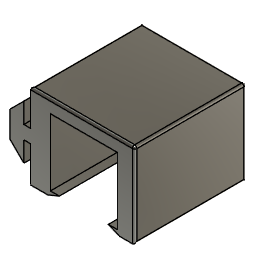
light bracket v2 (Autodesk Fusion 360 design; units mm, degrees)
Autodesk Fusion 360 part; units mm, degrees
sketch "Sketch1" plane through (0, 0, 0) normal (0, 0, 1) x (1, 0, 0) in component "Light Braccket"
  line L0 (0, 0) -> (-25, 0)
  line L1 (-25, 0) -> (-25, 25)
  line L2 (-25, 25) -> (0, 25)
  line L3 (0, 25) -> (0, 0)
  dimension "d1" = 25
  dimension "d2" = 25
  constraint horizontal L0
  constraint vertical L1
  constraint horizontal L2
  constraint vertical L3
  constraint coincident L0.start L3.end
  measures "d1" distance of L0.start L0.end
  measures "d2" distance of L0.start L2.end
extrude "Extrude1" add sketch "Sketch1" along normal blind 25 in component "Light Braccket"
sketch "Sketch2" plane through (0, 0, 0) normal (0, -1, 0) x (1, 0, 0) in component "Light Braccket"
  line L0 (-25, 0) -> (0, 0)
  line L1 (0, 0) -> (0, 25)
  line L2 (0, 25) -> (-25, 25)
  line L3 (-25, 25) -> (-25, 0)
  line L4 (-0.3536, 0) -> (-2.9142, 1.0607)
  line L5 (-0.3536, 0) -> (0.9236, 0) construction
  line L6 (-2.9142, 1.0607) -> (-0.9142, 1.0607)
  line L7 (-0.9142, 1.0607) -> (-0.9142, 16.0607)
  line L8 (-0.9142, 18.8102) -> (-15.9142, 18.8102) construction
  line L9 (-8.4142, 18.8102) -> (-8.4142, -0.114) construction
  line L10 (-16.4749, 0) -> (-13.9142, 1.0607)
  line L11 (-13.9142, 1.0607) -> (-15.9142, 1.0607)
  line L12 (-15.9142, 1.0607) -> (-15.9142, 16.0607)
  line L13 (-0.9142, 16.0607) -> (-15.9142, 16.0607)
  dimension "d14" = 15
  constraint horizontal L5
  constraint horizontal L6
  constraint perpendicular L6 L7
  constraint coincident L7 L8.start
  constraint perpendicular L7 L8
  constraint midpoint L8 L9.start
  constraint perpendicular L0 L9
  constraint symmetric L4.start L9 L10.start
  constraint symmetric L4.end L9 L10.end
  constraint symmetric L6.end L9 L11.end
  constraint symmetric L7.end L9 L12.end
  constraint perpendicular L12 L13
  measures "d14" distance of L8.start L8.end
extrude "Extrude2" cut sketch "Sketch2" against normal blind 40 contours L0 L4 L6 L7 L10 L11 L12 L13 in component "Light Braccket"
sketch "Sketch3" plane through (0, 0, 0) normal (0, -1, 0) x (1, 0, 0) in component "Light Braccket"
  line L0 (-16.4749, 0) -> (-13.9142, 1.0607)
  line L1 (-13.9142, 1.0607) -> (-15.9142, 1.0607)
  line L2 (-15.9142, 1.0607) -> (-15.9142, 16.0607)
  line L3 (-15.9142, 16.0607) -> (-0.9142, 16.0607)
  line L4 (-0.9142, 16.0607) -> (-0.9142, 1.0607)
  line L5 (-0.9142, 1.0607) -> (-2.9142, 1.0607)
  line L6 (-2.9142, 1.0607) -> (-0.3536, 0)
  line L7 (-0.3536, 0) -> (0, 0)
  line L8 (0, 0) -> (0, 25)
  line L9 (0, 25) -> (-25, 25)
  line L10 (-25, 25) -> (-25, 0)
  line L11 (-25, 0) -> (-16.4749, 0)
  line L12 (-25, 25) -> (0, 25)
  line L13 (0, 25) -> (0, 19)
  line L14 (0, 19) -> (-25, 19)
  line L15 (-25, 19) -> (-25, 25)
  constraint horizontal L12
  constraint vertical L13
  constraint horizontal L14
  constraint vertical L15
  constraint coincident L8 L13.end
  constraint coincident L9.end L10.start
extrude "Extrude3" cut sketch "Sketch3" against normal blind 39 contours L8 L9 L10 L12 L13 L14 L15 in component "Light Braccket"
sketch "Sketch4" plane through (0, 0, 0) normal (0, -1, 0) x (1, 0, 0) in component "Light Braccket"
  line L0 (0, 19) -> (-25, 19)
  line L1 (-25, 19) -> (-25, 0)
  line L2 (-25, 0) -> (-16.4749, 0)
  line L3 (-16.4749, 0) -> (-13.9142, 1.0607)
  line L4 (-13.9142, 1.0607) -> (-15.9142, 1.0607)
  line L5 (-15.9142, 1.0607) -> (-15.9142, 16.0607)
  line L6 (-15.9142, 16.0607) -> (-0.9142, 16.0607)
  line L7 (-0.9142, 16.0607) -> (-0.9142, 1.0607)
  line L8 (-0.9142, 1.0607) -> (-2.9142, 1.0607)
  line L9 (-2.9142, 1.0607) -> (-0.3536, 0)
  line L10 (-0.3536, 0) -> (0, 0)
  line L11 (0, 0) -> (0, 19)
  line L12 (-25, 0) -> (-25, 6.6)
  line L13 (-25, 6.6) -> (-21.8712, 3.4712)
  line L14 (-25, 6.6) -> (-20.5752, 6.6) construction
  line L15 (-21.8712, 3.4712) -> (-21.8712, 8)
  line L16 (-21.8712, 8) -> (-20.3712, 8)
  line L17 (-20.3712, 8) -> (-20.3712, 0)
  line L18 (-25, 0) -> (-20.3712, 0)
  line L19 (-25, 9.5) -> (0, 9.5) construction
  line L20 (-25, 12.4) -> (-21.8712, 15.5288)
  line L21 (-21.8712, 15.5288) -> (-21.8712, 11)
  line L22 (-20.3712, 11) -> (-20.3712, 19)
  line L23 (-21.8712, 11) -> (-20.3712, 11)
  line L24 (-25, 19) -> (-20.3712, 19)
  line L25 (-25, 19) -> (-25, 12.4)
  dimension "d19" = 6.6
  dimension "d20" = 45
  dimension "d21" = 1.5
  constraint coincident L1.end L2.start
  constraint perpendicular L0 L12
  constraint horizontal L14
  constraint perpendicular L14 L15
  constraint perpendicular L15 L16
  constraint coincident L2 L17.end
  constraint perpendicular L2 L17
  constraint midpoint L1 L19.start
  constraint midpoint L11 L19.end
  constraint symmetric L1.end L19 L0.end
  constraint symmetric L12.end L19 L20.start
  constraint symmetric L13.end L19 L20.end
  constraint symmetric L15.end L19 L21.end
  constraint symmetric L16.end L19 L22.start
  constraint symmetric L17.end L19 L22.end
  measures "d19" distance of L1.end L12.end
  measures "d20" angle of L13 L14
  measures "d21" distance of L15.end L16.end
extrude "Extrude4" cut sketch "Sketch4" against normal blind 33.5 contours L0 L1 L20 L21 L22 L23 L24 L25 | L1 L2 L12 L13 L15 L16 L17 L18 in component "Light Braccket"
sketch "Sketch1 (2)" plane through (0, 0, 0) normal (1, 0, 0) x (0, 1, 0)
  line L0 (25, 19) -> (0, 19)
  line L1 (0, 19) -> (0, 0)
  line L2 (0, 0) -> (25, 0)
  line L3 (25, 0) -> (25, 19)
extrude "Extrude5" add sketch "Sketch1 (2)" along normal blind 3 in component "Light Braccket"
fillet "Fillet2" radius 0.5 7 edges at (-8.6856, 0, 19) (-20.3712, 12.5, 19) (-8.6856, 25, 19) (3, 12.5, 19) (3, 0, 9.5) (3, 25, 9.5) (3, 12.5, 0) in component "Light Braccket"
component "Light Braccket" placed x (1, 0, 0) y (0, 1, 0) z (0, 0, 1) at (0, 0, 0)
